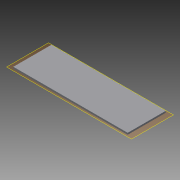
# Autodesk Inventor part: Syringe PCB
Saved by Autodesk Inventor 2015 SP1 (Build 190203100, 203)
## iProperties
Created: 2016-08-29
Part Number: Syringe PCB
Material: Generic
Document SubType Name: Modeling
Designer: lustinga
Density: 1 g/cm^3
Appearance: Default
Author: lustinga
Autodesk Inventor part; units mm, degrees
ref_plane "YZ Plane" through (0, 0, 0) normal (1, 0, 0) x (0, 1, 0)
ref_plane "XZ Plane" through (0, 0, 0) normal (0, 1, 0) x (-1, 0, 0)
ref_plane "XY Plane" through (0, 0, 0) normal (0, 0, 1) x (1, 0, 0)
ref_plane "Work Plane1" through (0, 0, 0) normal (0, 0, 1) x (1, 0, 0)
sketch "Sketch1" plane through (0, 0, 0) normal (0, 0, 1) x (1, 0, 0)
  circle A0 centre (6.766, 15.49) radius 1.5875
  circle A1 centre (-7.234, 15.49) radius 1.5875
  line L0 (-34.544, 11.43) -> (-34.544, -11.43)
  line L1 (-34.544, -11.43) -> (34.036, -11.43)
  line L2 (34.036, -11.43) -> (34.036, 11.43)
  line L3 (-10.3543, 11.43) -> (-10.3543, 18.7046)
  line L4 (-10.3543, 18.7046) -> (9.7417, 18.7046)
  line L5 (9.7417, 18.7046) -> (9.7417, 11.43)
  line L6 (34.036, 11.43) -> (9.7417, 11.43)
  line L7 (-10.3543, 11.43) -> (-34.544, 11.43)
  point P0 (0, 0)
  dimension "d0" = 68.58
  dimension "d1" = 22.86
  dimension "d2" = 27.31
  dimension "d3" = 14
  dimension "d4" = 3.175
  dimension "d5" = 3.175
  dimension "d10" = 26.92
  constraints: 16 end point, 3 parallel, 3 perpendicular, 2 centre point, 1 horizontal, 1 vertical
  measures "d0" distance of L0.start L2.end
  measures "d1" distance of L1.end L2.end
  measures "d2" distance from line of A1.centre L0
  measures "d3" distance of A0.centre A1.centre
  measures "d4" diameter of A0
  measures "d5" diameter of A1
  measures "d10" distance from line of A1.centre L1
extrude "Extrusion1" add sketch "Sketch1" along normal blind 1
body "Solid1"
